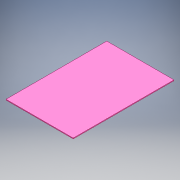
# Autodesk Inventor part: panel
Saved by Autodesk Inventor 2018 (Build 220112000, 112)
## iProperties
Created: 2018-01-24
Part Number: panel
Material: Generic
Document SubType Name: Modeling
Designer: mokuz
Density: 1 g/cm^3
Appearance: Pink
Author: mokuz
Autodesk Inventor part; units mm, degrees
ref_plane "YZ Plane" through (0, 0, 0) normal (1, 0, 0) x (0, 1, 0)
ref_plane "XZ Plane" through (0, 0, 0) normal (0, 1, 0) x (-1, 0, 0)
ref_plane "XY Plane" through (0, 0, 0) normal (0, 0, 1) x (1, 0, 0)
sketch "Sketch1" plane through (0, 0, 0) normal (0, 0, 1) x (1, 0, 0)
  line L0 (0, 0) -> (1400, 0)
  line L1 (1400, 0) -> (1400, 2100)
  line L2 (1400, 2100) -> (0, 2100)
  line L3 (0, 2100) -> (0, 0)
  dimension "d0" = 1400
  dimension "d1" = 2100
  constraints: 8 end point, 2 parallel, 1 horizontal, 1 perpendicular
  measures "d0" distance of L2.end L1.end
  measures "d1" distance of L1.end L0.end
extrude "Extrusion1" add sketch "Sketch1" along normal blind 16
body "Solid1"
